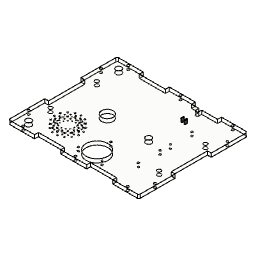
Carter_dessus_KOSMOS3-0 (Autodesk Fusion 360 design; units mm, degrees)
Autodesk Fusion 360 part; units mm, degrees
sketch "Esquisse1" plane through (0, 0, 0) normal (0, 0, 1) x (1, 0, 0)
  circle A0 centre (-16.5, 75) radius 3.95
  circle A1 centre (-73.5, 75) radius 8
  arc A2 (-133, 150) -> (-135, 148) centre (-133, 148) ccw
  arc A3 (43, 0) -> (45, 2) centre (43, 2) ccw
  arc A4 (45, 148) -> (43, 150) centre (43, 148) ccw
  arc A5 (-135, 2) -> (-133, 0) centre (-133, 2) ccw
  circle A6 centre (-37.6915, 25) radius 15.2
  line L0 (-135, 75) -> (45, 75) construction
  circle A7 centre (-73.5, 75) radius 61.5 construction
  line L1 (-45, 75) -> (-133, 148) construction
  circle A8 centre (-120, 12.7841) radius 3.95
  line L2 (-37.6915, 25) -> (-37.6915, 48) construction
  circle A9 centre (-37.6915, 44) radius 1.275
  circle A10 centre (-54.146, 15.5) radius 1.275
  circle A11 centre (-21.237, 15.5) radius 1.275
  line L3 (-99, 0) -> (-99, 5.3)
  line L4 (-99, 5.3) -> (-63, 5.3)
  line L5 (-63, 5.3) -> (-63, 0)
  line L6 (9, 0) -> (9, 5.3)
  line L7 (9, 5.3) -> (-27, 5.3)
  line L8 (-27, 5.3) -> (-27, 0)
  line L9 (-133, 0) -> (-99, 0)
  line L10 (-63, 0) -> (-27, 0)
  line L11 (9, 0) -> (43, 0)
  circle A12 centre (-45, 2.65) radius 1.5
  circle A13 centre (27, 2.65) radius 1.6
  line L12 (-63, 150) -> (-63, 144.7)
  line L13 (-63, 144.7) -> (-99, 144.7)
  line L14 (-99, 144.7) -> (-99, 150)
  line L15 (9, 150) -> (9, 144.7)
  line L16 (9, 144.7) -> (-27, 144.7)
  line L17 (-27, 144.7) -> (-27, 150)
  line L18 (-133, 150) -> (-99, 150)
  line L19 (-63, 150) -> (-27, 150)
  line L20 (9, 150) -> (43, 150)
  circle A14 centre (-45, 147.35) radius 1.5
  circle A15 centre (27, 147.35) radius 1.6
  line L21 (-135, 50) -> (-129.7, 50)
  line L22 (-129.7, 50) -> (-129.7, 100)
  line L23 (-129.7, 100) -> (-135, 100)
  line L24 (-135, 148) -> (-135, 100)
  line L25 (-135, 2) -> (-135, 50)
  line L26 (45, 100) -> (39.7, 100)
  line L27 (39.7, 100) -> (39.7, 50)
  line L28 (39.7, 50) -> (45, 50)
  line L29 (45, 148) -> (45, 100)
  line L30 (45, 2) -> (45, 50)
  circle A16 centre (-132.35, 125) radius 1.5
  circle A17 centre (-132.1585, 25) radius 1.5
  circle A18 centre (42.35, 125) radius 1.5
  circle A19 centre (42.35, 25) radius 1.5
  circle A20 centre (-117, 2.65) radius 1.6
  circle A21 centre (-120, 137.2159) radius 3.95
  circle A22 centre (-117, 147.35) radius 1.6
  circle A23 centre (6.309, 38) radius 1.275
  circle A24 centre (6.309, 68) radius 1.275
  circle A25 centre (6.309, 82) radius 1.275
  circle A26 centre (6.309, 112) radius 1.275
  point P0 (-135, 0)
  point P1 (-135, 150)
  point P2 (45, 150)
  dimension "d1" = 180
  dimension "d2" = 150
  dimension "d5" = 7.9
  dimension "d6" = 16
  dimension "d7" = 2
  dimension "d8" = 2
  dimension "d9" = 2
  dimension "d47" = 30.4
  dimension "d51" = 50
  dimension "d52" = 123
  dimension "d62" = 2.55
  dimension "d63" = 19
  dimension "d65" = 360
  dimension "d71" = 5.3
  dimension "d73" = 36
  dimension "d74" = 36
  dimension "d75" = 5.3
  dimension "d76" = 36
  dimension "d80" = 3
  dimension "d81" = 2.65
  dimension "d82" = 18
  dimension "d83" = 3.2
  dimension "d84" = 18
  dimension "d85" = 2.65
  dimension "d86" = 5.3
  dimension "d87" = 5.3
  dimension "d88" = 36
  dimension "d89" = 36
  dimension "d91" = 36
  dimension "d92" = 5.3
  dimension "d93" = 50
  dimension "d94" = 50
  dimension "d95" = 50
  dimension "d96" = 50
  dimension "d97" = 5.3
  dimension "d98" = 3
  dimension "d99" = 2.65
  dimension "d100" = 25
  dimension "d101" = 3
  dimension "d102" = 25
  dimension "d103" = 3
  dimension "d104" = 2.65
  dimension "d106" = 3
  dimension "d107" = 25
  dimension "d108" = 2.65
  dimension "d109" = 3.2
  dimension "d110" = 18
  dimension "d111" = 2.65
  dimension "d113" = 25
  dimension "d141" = 2.55
  dimension "d142" = 32.7
  dimension "d143" = 38.691
  dimension "d144" = 2.55
  dimension "d145" = 38.691
  dimension "d146" = 30
  constraint equal A2 A3
  constraint concentric A1 A7
  constraint coincident A6.centre A7
  constraint midpoint L0 L1.start
  constraint coincident A2.centre L1.end
  constraint coincident A6.centre L2.start
  constraint vertical L2
  constraint coincident L2 A9.centre
  constraint perpendicular L3 L4
  constraint vertical L6
  constraint horizontal L7
  constraint vertical L8
  constraint tangent A5 L9
  constraint perpendicular L8 L10
  constraint tangent A3 L11
  constraint vertical L12
  constraint horizontal L13
  constraint vertical L14
  constraint vertical L15
  constraint horizontal L16
  constraint vertical L17
  constraint tangent A2 L18
  constraint perpendicular L17 L19
  constraint tangent A4 L20
  constraint symmetric L0 A12 A14
  constraint symmetric L0 A13 A15
  constraint horizontal L21
  constraint vertical L22
  constraint horizontal L23
  constraint tangent A2 L24
  constraint tangent A5 L25
  constraint horizontal L26
  constraint vertical L27
  constraint horizontal L28
  constraint tangent A4 L29
  constraint tangent A3 L30
  constraint symmetric L0 A8 A21
  constraint symmetric L0 A20 A22
  constraint symmetric L0 A23 A26
  constraint symmetric L0 A24 A25
  measures "d1" distance of P1 P2
  measures "d2" distance of P0 P1
  measures "d5" diameter of A0
  measures "d6" diameter of A1
  measures "d7" radius of A2
  measures "d8" radius of A4
  measures "d9" radius of A5
  measures "d47" diameter of A6
  measures "d51" distance of A6.centre L0
  measures "d52" diameter of A7
  measures "d62" diameter of A9
  measures "d63" distance of A6.centre A9.centre
  measures "d71" distance of L3.start L3.end
  measures "d73" distance of L3.end L4.end
  measures "d74" distance of L8.end L6.start
  measures "d75" distance of L8.end L7.end
  measures "d76" distance of L5 L8
  measures "d80" diameter of A12
  measures "d81" distance of L10 A12.centre
  measures "d82" distance of L5 A12.centre
  measures "d83" diameter of A13
  measures "d84" distance of L6 A13.centre
  measures "d85" distance of L11 A13.centre
  measures "d86" distance of L14.end L13.end
  measures "d87" distance of L17.end L16.end
  measures "d88" distance of L12.end L13.end
  measures "d89" distance of L15.end L16.end
  measures "d91" distance of L12 L17
  measures "d92" distance of L21.start L21.end
  measures "d93" distance of L9 L21
  measures "d94" distance of L21.end L22.end
  measures "d95" distance of L20 L26
  measures "d96" distance of L26.end L27.end
  measures "d97" distance of L26.start L26.end
  measures "d98" diameter of A16
  measures "d99" distance of L24 A16.centre
  measures "d100" distance of L23 A16.centre
  measures "d101" diameter of A17
  measures "d102" distance of L21 A17.centre
  measures "d103" diameter of A18
  measures "d104" distance of L29 A18.centre
  measures "d106" diameter of A19
  measures "d107" distance of L28 A19.centre
  measures "d108" distance of L30 A19.centre
  measures "d109" diameter of A20
  measures "d110" distance of L3 A20.centre
  measures "d111" distance of L9 A20.centre
  measures "d113" distance of L26 A18.centre
  measures "d141" diameter of A23
  measures "d142" distance of L7 A23.centre
  measures "d143" distance of L30 A23.centre
  measures "d144" diameter of A24
  measures "d145" distance of L30 A24.centre
  measures "d146" distance of A23.centre A24.centre
extrude "Extrusion1" add sketch "Esquisse1" along normal blind 5
sketch "Esquisse2" plane through (0, 0, 5) normal (0, 0, 1) x (-1, 0, 0)
  circle A0 centre (73.5, -75) radius 8
  circle A1 centre (16.5, -75) radius 3.95
  arc A2 (133, -150) -> (135, -148) centre (133, -148) ccw
  arc A3 (135, -2) -> (133, 0) centre (133, -2) ccw
  arc A4 (-43, 0) -> (-45, -2) centre (-43, -2) ccw
  arc A5 (-45, -148) -> (-43, -150) centre (-43, -148) ccw
  line L0 (135, -75) -> (-45, -75) construction
  line L1 (120, -75) -> (120, -150) construction
  line L2 (45, -150) -> (45, 0) construction
  circle A6 centre (37.6915, -25) radius 15.2
  circle A7 centre (120, -12.7841) radius 3.95
  circle A8 centre (37.6915, -44) radius 1.275
  circle A9 centre (54.146, -15.5) radius 1.275
  circle A10 centre (21.237, -15.5) radius 1.275
  circle A11 centre (120, -107) radius 2.6
  circle A12 centre (120, -43) radius 2.6
  circle A13 centre (-30, -43) radius 2.6
  circle A14 centre (-30, -107) radius 2.6
  line L3 (-9, -5.3) -> (-9, 0)
  line L4 (-9, 0) -> (-43, 0)
  line L5 (133, 0) -> (99, 0)
  line L6 (99, 0) -> (99, -5.3)
  line L7 (99, -5.3) -> (63, -5.3)
  line L8 (63, -5.3) -> (63, 0)
  line L9 (63, 0) -> (27, 0)
  line L10 (27, 0) -> (27, -5.3)
  line L11 (27, -5.3) -> (-9, -5.3)
  line L12 (-9, -144.7) -> (27, -144.7)
  line L13 (27, -144.7) -> (27, -150)
  line L14 (27, -150) -> (63, -150)
  line L15 (63, -150) -> (63, -144.7)
  line L16 (63, -144.7) -> (99, -144.7)
  line L17 (99, -144.7) -> (99, -150)
  line L18 (99, -150) -> (133, -150)
  line L19 (-43, -150) -> (-9, -150)
  line L20 (-9, -150) -> (-9, -144.7)
  line L21 (-45, -2) -> (-45, -50)
  line L22 (-45, -50) -> (-39.7, -50)
  line L23 (-39.7, -50) -> (-39.7, -100)
  line L24 (-39.7, -100) -> (-45, -100)
  line L25 (-45, -100) -> (-45, -148)
  line L26 (135, -148) -> (135, -100)
  line L27 (135, -100) -> (129.7, -100)
  line L28 (129.7, -100) -> (129.7, -50)
  line L29 (129.7, -50) -> (135, -50)
  line L30 (135, -50) -> (135, -2)
  circle A15 centre (-27, -2.65) radius 1.6
  circle A16 centre (45, -2.65) radius 1.5
  circle A17 centre (45, -147.35) radius 1.5
  circle A18 centre (-42.35, -25) radius 1.5
  circle A19 centre (-42.35, -125) radius 1.5
  circle A20 centre (132.1585, -25) radius 1.5
  circle A21 centre (-27, -147.35) radius 1.6
  circle A22 centre (132.35, -125) radius 1.5
  circle A23 centre (120, -137.2159) radius 3.95
  circle A24 centre (117, -147.35) radius 1.6
  circle A25 centre (117, -2.65) radius 1.6
  circle A26 centre (-6.309, -38) radius 1.275
  circle A27 centre (-6.309, -68) radius 1.275
  circle A28 centre (-6.309, -112) radius 1.275
  circle A29 centre (-6.309, -82) radius 1.275
  point P0 (-30, -75)
  dimension "d53" = 16
  dimension "d66" = 5.2
  dimension "d69" = 32
  dimension "d70" = 75
  constraint coincident L0 L1.start
  constraint symmetric L1.start L2 P0
  constraint coincident L1 A11.centre
  constraint symmetric L0 A11 A12
  constraint symmetric L2 A12 A13
  constraint symmetric L2 A11 A14
  constraint midpoint L0 L2
  measures "d53" diameter of A0
  measures "d66" diameter of A11
  measures "d69" distance of L0 A11.centre
  measures "d70" distance of L1 L2
extrude "Extrusion4" cut sketch "Esquisse2" against normal blind 5 contours A11 | A12 | A13 | A14
sketch "Esquisse3" plane through (0, 0, 5) normal (0, 0, 1) x (-1, 0, 0)
  circle A0 centre (120, -43) radius 2.6
  circle A1 centre (-30, -43) radius 2.6
  circle A2 centre (120, -107) radius 2.6
  circle A3 centre (-30, -107) radius 2.6
  circle A4 centre (37.6915, -25) radius 15.2
  circle A5 centre (-42.35, -125) radius 1.5
  circle A6 centre (37.6915, -44) radius 1.275
  circle A7 centre (16.5, -75) radius 3.95
  circle A8 centre (54.146, -15.5) radius 1.275
  circle A9 centre (117, -2.65) radius 1.6
  circle A10 centre (21.237, -15.5) radius 1.275
  circle A11 centre (117, -147.35) radius 1.6
  circle A12 centre (-42.35, -25) radius 1.5
  circle A13 centre (120, -12.7841) radius 3.95
  circle A14 centre (-27, -147.35) radius 1.6
  circle A15 centre (45, -2.65) radius 1.5
  circle A16 centre (-27, -2.65) radius 1.6
  circle A17 centre (45, -147.35) radius 1.5
  circle A18 centre (132.1585, -25) radius 1.5
  circle A19 centre (132.35, -125) radius 1.5
  circle A20 centre (120, -137.2159) radius 3.95
  circle A21 centre (73.5, -75) radius 8
  line L0 (-9, 0) -> (-43, 0)
  arc A22 (-43, 0) -> (-45, -2) centre (-43, -2) ccw
  line L1 (-45, -2) -> (-45, -50)
  line L2 (-45, -50) -> (-39.7, -50)
  line L3 (-39.7, -50) -> (-39.7, -100)
  line L4 (-39.7, -100) -> (-45, -100)
  line L5 (-45, -100) -> (-45, -148)
  arc A23 (-45, -148) -> (-43, -150) centre (-43, -148) ccw
  line L6 (-43, -150) -> (-9, -150)
  line L7 (-9, -150) -> (-9, -144.7)
  line L8 (-9, -144.7) -> (27, -144.7)
  line L9 (27, -144.7) -> (27, -150)
  line L10 (27, -150) -> (63, -150)
  line L11 (63, -150) -> (63, -144.7)
  line L12 (63, -144.7) -> (99, -144.7)
  line L13 (99, -144.7) -> (99, -150)
  line L14 (99, -150) -> (133, -150)
  arc A24 (133, -150) -> (135, -148) centre (133, -148) ccw
  line L15 (135, -148) -> (135, -100)
  line L16 (135, -100) -> (129.7, -100)
  line L17 (129.7, -100) -> (129.7, -50)
  line L18 (129.7, -50) -> (135, -50)
  line L19 (135, -50) -> (135, -2)
  arc A25 (135, -2) -> (133, 0) centre (133, -2) ccw
  line L20 (133, 0) -> (99, 0)
  line L21 (99, 0) -> (99, -5.3)
  line L22 (99, -5.3) -> (63, -5.3)
  line L23 (63, -5.3) -> (63, 0)
  line L24 (63, 0) -> (27, 0)
  line L25 (27, 0) -> (27, -5.3)
  line L26 (27, -5.3) -> (-9, -5.3)
  line L27 (-9, -5.3) -> (-9, 0)
  line L28 (133, -2) -> (-43, -148) construction
  circle A26 centre (90.41, -37.3303) radius 17.5 construction
  circle A27 centre (101.2616, -23.6011) radius 1
  circle A28 centre (94.7392, -20.3743) radius 1
  circle A29 centre (87.4683, -20.0794) radius 1
  circle A30 centre (80.706, -22.7673) radius 1
  circle A31 centre (75.6216, -27.9733) radius 1
  circle A32 centre (73.0943, -34.7972) radius 1
  circle A33 centre (73.561, -42.0592) radius 1
  circle A34 centre (76.9411, -48.5034) radius 1
  circle A35 centre (82.65, -53.0158) radius 1
  circle A36 centre (89.7008, -54.816) radius 1
  circle A37 centre (96.8741, -53.5927) radius 1
  circle A38 centre (102.9298, -49.5576) radius 1
  circle A39 centre (106.8206, -43.4082) radius 1
  circle A40 centre (107.874, -36.208) radius 1
  circle A41 centre (105.9076, -29.2018) radius 1
  circle A42 centre (90.41, -37.3303) radius 14 construction
  circle A43 centre (96.618, -24.782) radius 0.8
  line L29 (101.2616, -23.6011) -> (90.41, -37.3303) construction
  line L30 (96.618, -24.782) -> (90.41, -37.3303) construction
  circle A44 centre (90.9774, -23.3418) radius 0.8
  circle A45 centre (85.2387, -24.3204) radius 0.8
  circle A46 centre (80.3942, -27.5485) radius 0.8
  circle A47 centre (77.2815, -32.468) radius 0.8
  circle A48 centre (76.4388, -38.2282) radius 0.8
  circle A49 centre (78.0119, -43.8332) radius 0.8
  circle A50 centre (81.7287, -48.3138) radius 0.8
  circle A51 centre (86.9466, -50.8952) radius 0.8
  circle A52 centre (92.7634, -51.1311) radius 0.8
  circle A53 centre (98.1732, -48.9808) radius 0.8
  circle A54 centre (102.2407, -44.816) radius 0.8
  circle A55 centre (104.2626, -39.3568) radius 0.8
  circle A56 centre (103.8892, -33.5473) radius 0.8
  circle A57 centre (101.1851, -28.3919) radius 0.8
  circle A58 centre (90.41, -37.3303) radius 10.5 construction
  circle A59 centre (96.921, -29.0928) radius 0.6
  circle A60 centre (93.0075, -27.1567) radius 0.6
  circle A61 centre (88.645, -26.9798) radius 0.6
  circle A62 centre (84.5876, -28.5925) radius 0.6
  circle A63 centre (81.537, -31.7161) radius 0.6
  circle A64 centre (80.0206, -35.8105) radius 0.6
  circle A65 centre (80.3006, -40.1676) radius 0.6
  circle A66 centre (82.3286, -44.0342) radius 0.6
  circle A67 centre (85.754, -46.7416) radius 0.6
  circle A68 centre (89.9845, -47.8217) radius 0.6
  circle A69 centre (94.2885, -47.0878) radius 0.6
  circle A70 centre (97.9219, -44.6667) radius 0.6
  circle A71 centre (100.2564, -40.9771) radius 0.6
  circle A72 centre (100.8884, -36.6569) radius 0.6
  circle A73 centre (99.7086, -32.4532) radius 0.6
  line L31 (45, -75) -> (53.0468, -84.7003) construction
  circle A74 centre (-6.309, -38) radius 1.275
  circle A75 centre (-6.309, -68) radius 1.275
  circle A76 centre (-6.309, -112) radius 1.275
  circle A77 centre (-6.309, -82) radius 1.275
  line L32 (17, -144.7) -> (13, -144.7)
  line L33 (13, -144.7) -> (13, -140.7)
  line L34 (15.0171, -138.7) -> (15.0171, -138.7)
  line L35 (17, -140.7) -> (17, -144.7)
  arc A78 (17, -140.7) -> (15, -138.7) centre (15, -140.7) ccw
  arc A79 (15, -138.7) -> (13, -140.7) centre (15, -140.7) ccw
  line L36 (15, -144.7) -> (15, -140.7) construction
  line L37 (15, -144.7) -> (15, -86.7887) construction
  line L38 (18, -120.7) -> (12, -120.7)
  line L39 (12, -121.2) -> (12, -124.2)
  line L40 (12, -124.7) -> (17.5, -124.7)
  line L41 (18, -124.2) -> (18, -121.2)
  line L42 (17.5, -120.7) -> (17, -120.7)
  line L43 (16.5, -121.2) -> (16.5, -124.2)
  line L44 (17, -124.7) -> (18, -124.7)
  line L45 (18, -124.7) -> (18, -120.7)
  line L46 (12.5, -120.7) -> (13, -120.7)
  line L47 (13.5, -121.2) -> (13.5, -124.2)
  line L48 (13, -124.7) -> (12.5, -124.7)
  line L49 (12, -124.7) -> (12, -120.7)
  arc A80 (17, -120.7) -> (16.5, -121.2) centre (17, -121.2) ccw
  arc A81 (18, -121.2) -> (17.5, -120.7) centre (17.5, -121.2) ccw
  arc A82 (17.5, -124.7) -> (18, -124.2) centre (17.5, -124.2) ccw
  arc A83 (16.5, -124.2) -> (17, -124.7) centre (17, -124.2) ccw
  arc A84 (13, -124.7) -> (13.5, -124.2) centre (13, -124.2) ccw
  arc A85 (13.5, -121.2) -> (13, -120.7) centre (13, -121.2) ccw
  arc A86 (12.5, -120.7) -> (12, -121.2) centre (12.5, -121.2) ccw
  arc A87 (12, -124.2) -> (12.5, -124.7) centre (12.5, -124.2) ccw
  point P0 (17, -138.7)
  point P1 (18, -124.7)
  point P2 (13.5, -120.7)
  dimension "d114" = 35
  dimension "d115" = 2
  dimension "d117" = 360
  dimension "d118" = 28
  dimension "d119" = 12
  dimension "d120" = 24
  dimension "d121" = 1.6
  dimension "d123" = 360
  dimension "d124" = 21
  dimension "d126" = 1.2
  dimension "d128" = 360
  dimension "d147" = 4
  dimension "d148" = 6
  dimension "d149" = 2
  dimension "d153" = 60
  dimension "d154" = 6
  dimension "d155" = 4
  dimension "d156" = 3
  dimension "d157" = 4
  dimension "d158" = 1.5
  dimension "d159" = 4
  dimension "d160" = 0.5
  dimension "d161" = 20
  constraint coincident A25.centre L28.start
  constraint coincident A23.centre L28.end
  constraint coincident L28 A26.centre
  constraint coincident A26 A27.centre
  constraint concentric A26 A42
  constraint coincident A42 A43.centre
  constraint coincident A27.centre L29.start
  constraint coincident A26.centre A42.centre
  constraint coincident A43.centre L30.start
  constraint concentric A42 A58
  constraint coincident A58 A59.centre
  constraint coincident L29 A59.centre
  constraint midpoint L28 L31.start
  constraint perpendicular L28 L31
  constraint horizontal L32
  constraint vertical L33
  constraint vertical L35
  constraint coincident L8 L32.start
  constraint coincident P0 L35
  constraint tangent L35 A78
  constraint tangent L33 A79
  constraint equal A78 A79
  constraint midpoint L32 L36.start
  constraint coincident A78.centre A79.centre
  constraint parallel L36 L37
  constraint horizontal L38
  constraint vertical L39
  constraint horizontal L40
  constraint vertical L41
  constraint horizontal L42
  constraint vertical L43
  constraint horizontal L44
  constraint vertical L45
  constraint horizontal L46
  constraint vertical L47
  constraint horizontal L48
  constraint vertical L49
  constraint tangent L42 A80
  constraint tangent L43 A80
  constraint coincident L38.start L42
  constraint coincident L38.start L41
  constraint tangent L42 A81
  constraint tangent L41 A81
  constraint equal A80 A81
  constraint coincident P1 L40
  constraint coincident P1 L41
  constraint tangent L40 A82
  constraint tangent L41 A82
  constraint equal A80 A82
  constraint tangent L44 A83
  constraint tangent L43 A83
  constraint equal A80 A83
  constraint tangent L48 A84
  constraint tangent L47 A84
  constraint equal A80 A84
  constraint coincident P2 L47
  constraint coincident P2 L46
  constraint tangent L47 A85
  constraint tangent L46 A85
  constraint equal A80 A85
  constraint coincident L38.end L39
  constraint coincident L38.end L46
  constraint tangent L39 A86
  constraint tangent L46 A86
  constraint equal A80 A86
  constraint coincident L40.start L39
  constraint coincident L40.start L48
  constraint tangent L39 A87
  constraint tangent L48 A87
  constraint equal A80 A87
  measures "d114" diameter of A26
  measures "d115" diameter of A27
  measures "d118" diameter of A42
  measures "d119" angle of L28 L29
  measures "d120" angle of L28 L30
  measures "d121" diameter of A43
  measures "d124" diameter of A58
  measures "d126" diameter of A59
  measures "d147" distance of L32.start L32.end
  measures "d148" distance of L32.start P0
  measures "d149" radius of A78
  measures "d153" distance of L5 L36
  measures "d154" distance of L38.start L38.end
  measures "d155" distance of L38.start P1
  measures "d156" distance of L37 L41
  measures "d157" distance of L38.start P1
  measures "d158" distance of L38.end P2
  measures "d159" distance of L38.end L40.start
  measures "d160" radius of A80
  measures "d161" distance of L8 L40
extrude "Extrusion5" cut sketch "Esquisse3" against normal blind 5 contours L8 L32 L33 L35 A78 A79 | A27 | A28 | A29 | A30 | A31 | A32 | A33 | A34 | A35 | A36 | A37 | A38 | A39 | A40 | A41 | A43 | A44 | A45 | A46 | A47 | A48 | A49 | A50 | A51 | A52 | A53 | A54 | A55 | A56 | A57 | A59 | A60 | A61 | A62 | A63 | A64 | A65 | A66 | A67 | A68 | A69 | A70 | A71 | A72 | A73 | L38 L40 L41 L42 L43 L44 L45 A80 A81 A82 A83 | L38 L39 L40 L46 L47 L48 L49 A84 A85 A86 A87
equation "d72 = 36 mm"
equation "d73 = d72"
equation "d74 = d76"
equation "d75 = d71"
equation "d76 = d73"
equation "d77 = 3 mm"
equation "d81 = d75 / 2"
equation "d82 = d76 / 2"
equation "d83 = d109"
equation "d84 = d74 / 2"
equation "d85 = d75 / 2"
equation "d86 = d71"
equation "d87 = d86"
equation "d88 = d72"
equation "d89 = d88"
equation "d91 = d88"
equation "d92 = d71"
equation "d95 = d94"
equation "d96 = d94"
equation "d97 = d71"
equation "d98 = d77"
equation "d99 = d92 / 2"
equation "d100 = d94 / 2"
equation "d101 = d77"
equation "d102 = d100"
equation "d103 = d98"
equation "d104 = d97 / 2"
equation "d106 = d103"
equation "d107 = d96 / 2"
equation "d108 = d97 / 2"
equation "d110 = d73 / 2"
equation "d111 = d71 / 2"
equation "d113 = d95 / 2"
equation "d144 = d141"
equation "d145 = d143"
equation "d156 = d154 / 2"
